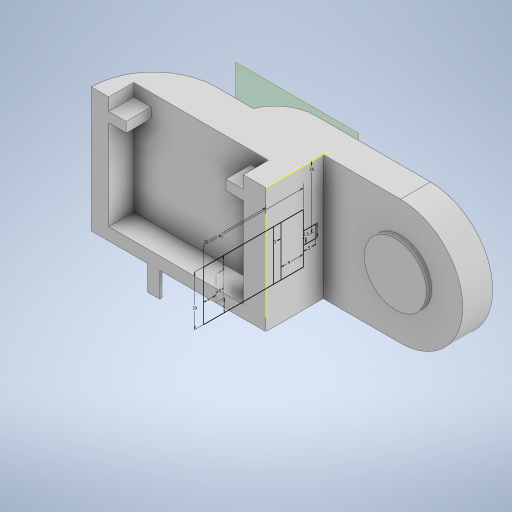
# Autodesk Inventor part: Part3
Saved by Autodesk Inventor 2023 (Build 270158000, 158)
## iProperties
Created: 2024-06-27
Part Number: Part3
Material: Generic
Document SubType Name: Modeling
Designer: Swoby
Density: 1 g/cm^3
Appearance: Default
Author: Swoby
Autodesk Inventor part; units mm, degrees
ref_plane "YZ Plane" through (0, 0, 0) normal (1, 0, 0) x (0, 1, 0)
ref_plane "XZ Plane" through (0, 0, 0) normal (0, 1, 0) x (-1, 0, 0)
ref_plane "XY Plane" through (0, 0, 0) normal (0, 0, 1) x (1, 0, 0)
sketch "Sketch1" plane through (0, 0, 0) normal (0, 1, 0) x (-1, 0, 0)
  arc A0 (0, -25) -> (25, 0) centre (0, 0) ccw
  line L0 (25, 0) -> (0, 0) construction
  line L1 (0, -25) -> (0, 0) construction
  arc A1 (25, 0) -> (-25, 0) centre (0, 0) ccw construction
  arc A2 (-25, 0) -> (0, -25) centre (0, 0) ccw construction
  line L2 (18, 10) -> (-36, 10)
  line L3 (-36, 10) -> (-36, -10)
  line L4 (-36, -10) -> (18, -10)
  line L5 (18, -10) -> (18, 10)
  line L6 (11, 10) -> (11, -10)
  line L7 (-29, 10) -> (-29, -10)
  line L8 (0, -25) -> (-45, -25)
  line L9 (-45, -25) -> (-45, 0)
  line L10 (-45, 0) -> (-36, 0)
  line L11 (25, 0) -> (18, 0)
  point P0 (11, 0)
  dimension "d0" = 50
  dimension "d1" = 20
  dimension "d2" = 10
  dimension "d3" = 54
  dimension "d4" = 7
  dimension "d5" = 7
  dimension "d7" = 11
  dimension "d8" = 45
  constraints: 24 end point, 6 point on circle, 5 perpendicular, 5 point on line, 3 centre point, 3 horizontal, 3 midpoint, 2 parallel, 1 coincident, 1 tangent, 1 vertical
  measures "d0" diameter of A0
  measures "d1" distance of L4.end L2.start
  measures "d2" distance from line of L4 point (0, 0)
  measures "d3" distance of L3.end L4.end
  measures "d4" distance between parallel lines of L6 L5
  measures "d5" distance between parallel lines of L3 L7
  measures "d7" distance of point (0, 0) point (11, 0)
  measures "d8" distance of L1.start L8.end
extrude "Extrusion1" add sketch "Sketch1" along normal blind 50 contours L8 L9 L10 L3 L4 L5 L11 A0
sketch "Sketch2" plane through (-18, 0, -10) normal (0, 0, 1) x (1, 0, 0)
  line L0 (7, 50) -> (7, 41) construction
  line L1 (7, 41) -> (0, 41) construction
  line L2 (0, 41) -> (0, 38) construction
  line L3 (0, 0) -> (0, 50) construction
  line L4 (0, 38) -> (7, 38) construction
  line L5 (7, 38) -> (7, 18) construction
  line L6 (7, 18) -> (2, 18) construction
  line L7 (2, 18) -> (2, 15) construction
  line L8 (2, 15) -> (7, 15) construction
  line L9 (7, 15) -> (7, 10) construction
  line L10 (7, 10) -> (47, 10) construction
  line L11 (47, 10) -> (47, 38) construction
  line L12 (47, 38) -> (54, 38) construction
  line L13 (54, 0) -> (54, 50) construction
  line L14 (54, 38) -> (54, 41) construction
  line L15 (54, 41) -> (47, 41) construction
  line L16 (47, 50) -> (20.5, 50) construction
  line L17 (20.5, 50) -> (20.5, 55) construction
  line L18 (20.5, 55) -> (15.5, 55) construction
  line L19 (15.5, 55) -> (15.5, 50) construction
  line L20 (15.5, 50) -> (7, 50) construction
  line L21 (47, 50) -> (47, 41) construction
  line L22 (0, 50) -> (54, 50) construction
  line L23 (7, 41) -> (0, 41)
  line L24 (0, 41) -> (0, 45)
  line L25 (0, 45) -> (7, 45)
  line L26 (7, 45) -> (7, 41)
  line L27 (47, 41) -> (54, 41)
  line L28 (54, 41) -> (54, 45)
  line L29 (54, 45) -> (47, 45)
  line L30 (47, 45) -> (47, 41)
  line L31 (0, 0) -> (0, 50) projected
  line L32 (0, 5) -> (54, 5)
  line L33 (54, 5) -> (54, 0)
  line L34 (54, 0) -> (0, 0)
  line L35 (0, 0) -> (0, 5)
  point P0 (18, 0)
  point P1 (4.5, 18)
  point P2 (3.5, 38)
  point P3 (18, 55)
  dimension "d11" = 40
  dimension "d12" = 3
  dimension "d13" = 3
  dimension "d16" = 9
  dimension "d17" = 5
  dimension "d18" = 5
  dimension "d19" = 7
  dimension "d20" = 7
  dimension "d21" = 5
  dimension "d22" = 5
  dimension "d23" = 11
  dimension "d24" = 4
  dimension "d29" = 5
  constraints: 64 end point, 18 point on line, 15 perpendicular, 6 parallel, 4 horizontal, 3 midpoint, 1 collinear
  measures "d11" distance between parallel lines of L10 L16
  measures "d12" distance between parallel lines of L4 L1
  measures "d13" distance from line of L8 point (4.5, 18)
  measures "d16" distance of L0.start L0.end
  measures "d17" distance between parallel lines of L10 L8
  measures "d18" distance of L5.end L6.end
  measures "d19" distance of L0.end L1.end
  measures "d20" distance of L14.end L15.end
  measures "d21" distance of L17.end L18.end
  measures "d22" distance of L16.end L17.end
  measures "d23" distance from line of L0 point (18, 55)
  measures "d24" distance between parallel lines of L1 L25
  measures "d29" distance between parallel lines of L34 L32
extrude "Extrusion2" add sketch "Sketch2" along normal up to surface (10 mm away)
sketch "Sketch4" plane through (0, 0, 0) normal (0, -1, 0) x (1, 0, 0)
  line L0 (-18, 0) -> (36, 0) projected
  circle A0 centre (0, 0) radius 2.5
  point P0 (2.5, 0)
  point P1 (-2.5, 0)
  dimension "d31" = 5
  constraints: 1 centre point, 1 coincident
  measures "d31" diameter of A0
extrude "Extrusion3" add sketch "Sketch4" along normal blind 10 contours L0 A0 picked at (-0.4734, -0.6858)
sketch "Sketch5" plane through (45, 0, 0) normal (1, 0, 0) x (0, 0, -1)
  line L0 (15, 35) -> (-25, 35)
  line L1 (-25, 35) -> (-25, 15)
  line L2 (-25, 15) -> (15, 15)
  line L3 (15, 15) -> (15, 35)
  line L4 (6, 35) -> (6, 15)
  line L5 (3, 35) -> (3, 15)
  line L6 (-17, 30) -> (-20, 30) construction
  line L7 (-20, 30) -> (-20, 20) construction
  line L8 (-20, 20) -> (-17, 20) construction
  line L9 (-17, 20) -> (-17, 30) construction
  line L10 (0, 5) -> (0, 41) projected
  line L11 (15, 27.5) -> (20, 27.5)
  line L12 (20, 27.5) -> (20, 22.5)
  line L13 (20, 22.5) -> (15, 22.5)
  line L14 (0, 50) -> (25, 50) projected
  point P0 (0, 0)
  point P1 (15, 25)
  dimension "d34" = 20
  dimension "d35" = 5
  dimension "d36" = 5
  dimension "d37" = 5
  dimension "d38" = 3
  dimension "d39" = 40
  dimension "d40" = 9
  dimension "d41" = 3
  dimension "d42" = 25
  dimension "d43" = 5
  dimension "d44" = 5
  dimension "d45" = 2.5
  dimension "d48" = 25
  constraints: 26 end point, 6 perpendicular, 6 point on line, 4 parallel, 3 horizontal, 1 midpoint
  measures "d34" distance of L0.end L1.end
  measures "d35" distance between parallel lines of L2 L8
  measures "d36" distance between parallel lines of L0 L6
  measures "d37" distance between parallel lines of L1 L7
  measures "d38" distance between parallel lines of L7 L9
  measures "d39" distance between parallel lines of L1 L3
  measures "d40" distance from line of point (15, 25) L4
  measures "d41" distance between parallel lines of L5 L4
  measures "d42" distance between parallel lines of L1 L10
  measures "d43" distance of L11.end L12.end
  measures "d44" distance of L12.end L13.end
  measures "d45" distance from line of L13 point (15, 25)
  measures "d48" distance from line of L14 point (15, 25)
ref_plane "Work Plane1" through (45, 0, -35) normal (0, 0, -1) x (-1, 0, 0)
sketch "Sketch6" plane through (45, 0, -35) normal (0, 0, -1) x (-1, 0, 0)
  circle A0 centre (-31, 25) radius 12.5
  circle A1 centre (-31, 25) radius 25
  line L0 (0, 0) -> (0, 50) projected
  line L1 (0, 25) -> (-26, 25) construction
  line L2 (-31, 50) -> (0, 50)
  line L3 (0, 0) -> (45, 0) projected
  line L4 (0, 0) -> (-31, 0)
  point P0 (0, 25)
  dimension "d50" = 25
  dimension "d51" = 50
  dimension "d52" = 31
  constraints: 6 end point, 2 centre point, 2 point on circle, 2 point on line, 1 coincident, 1 horizontal, 1 midpoint, 1 perpendicular, 1 tangent
  measures "d50" diameter of A0
  measures "d51" diameter of A1
  measures "d52" distance from line of L0 A0.centre
extrude "Extrusion4" add sketch "Sketch6" against normal blind 12 contours A0 | A1 | A1 L2 L0 L4
sketch "Sketch7" plane through (0, 50, 0) normal (0, 1, 0) x (1, 0, 0)
  arc A0 (0, 25) -> (-25, 0) centre (0, 0) ccw projected
  line L0 (-18, 0) -> (36, 0) projected
  line L1 (-25, 0) -> (-18, 0) projected
  line L2 (45, 35) -> (45, 25) projected
  line L3 (45, 35) -> (30, 35)
  line L4 (45, 25) -> (0, 25) projected
  arc A1 (30, 35) -> (15, 25) centre (30, 18.75) ccw
  dimension "d56" = 15
  dimension "d59" = 15
  dimension "d60" = 10
  constraints: 3 end point, 2 point on circle, 1 centre point, 1 perpendicular, 1 point on line, 1 tangent
  measures "d56" distance of L4.end A1.end
  measures "d59" horizontal distance of A1.centre A1.end
  measures "d60" distance between parallel lines of L4 L3
extrude "Extrusion5" add sketch "Sketch7" against normal up to surface (50 mm away)
sketch "Sketch8" plane through (45, 0, -23) normal (0, 0, 1) x (1, 0, 0)
  circle A0 centre (31, 25) radius 12.5
  arc A1 (31, 0) -> (31, 50) centre (31, 25) ccw projected
  point P0 (-45, 0)
  dimension "d63" = 25
  constraints: 1 centre point, 1 coincident
  measures "d63" diameter of A0
extrude "Extrusion6" add sketch "Sketch8" along normal blind 2
equation "\"d59\" = 1.5 * d60"
body "Solid1"
